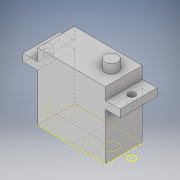
# Autodesk Inventor part: micro_servo
Saved by Autodesk Inventor 2018 (Build 220112000, 112)
## iProperties
Created: 2018-04-21
Part Number: micro_servo
Material: Generic
Document SubType Name: Modeling
Designer: scwu
Density: 1 g/cm^3
Appearance: Default
Author: scwu
Autodesk Inventor part; units mm, degrees
ref_plane "YZ Plane" through (0, 0, 0) normal (1, 0, 0) x (0, 1, 0)
ref_plane "XZ Plane" through (0, 0, 0) normal (0, 1, 0) x (-1, 0, 0)
ref_plane "XY Plane" through (0, 0, 0) normal (0, 0, 1) x (1, 0, 0)
sketch "Sketch1" plane through (0, 0, 0) normal (0, 0, 1) x (1, 0, 0)
  line L0 (-11.25, 0) -> (11.25, 0)
  line L1 (11.25, 0) -> (11.25, 15.72)
  line L2 (11.25, 15.72) -> (16.13, 15.72)
  line L3 (16.13, 15.72) -> (16.13, 18.22)
  line L4 (16.13, 18.22) -> (11.25, 18.22)
  line L5 (11.25, 18.22) -> (11.25, 22.22)
  line L6 (11.25, 22.22) -> (-11.25, 22.22)
  line L7 (-11.25, 22.22) -> (-11.25, 18.22)
  line L8 (-11.25, 18.22) -> (-16.13, 18.22)
  line L9 (-16.13, 18.22) -> (-16.13, 15.72)
  line L10 (-16.13, 15.72) -> (-11.25, 15.72)
  line L11 (-11.25, 0) -> (-11.25, 15.72)
  point P0 (0, 0)
  point P1 (0, 0)
  dimension "d0" = 22.5
  dimension "d1" = 15.72
  dimension "d2" = 4.88
  dimension "d3" = 2.5
  dimension "d4" = 4
  dimension "d5" = 4.88
  constraints: 24 end point, 8 perpendicular, 7 point on line, 1 coincident, 1 horizontal, 1 midpoint
  measures "d0" distance of L0.start L0.end
  measures "d1" distance of L0.end L1.end
  measures "d2" distance of L1.end L2.end
  measures "d3" distance of L2.end L3.end
  measures "d4" distance of L4.end L5.end
  measures "d5" distance of L7.end L8.end
extrude "Extrusion1" add sketch "Sketch1" along normal mid plane 12.23
sketch "Sketch2" plane through (-16.13, 18.22, 6.115) normal (0, 1, 0) x (1, 0, 0)
  line L0 (4.88, 12.23) -> (4.88, 0) projected
  line L1 (27.38, 0) -> (4.88, 0) projected
  line L2 (27.38, 12.23) -> (27.38, 0) projected
  line L3 (4.88, 12.23) -> (27.38, 12.23) projected
  line L4 (27.38, 0) -> (4.88, 0) projected
  line L5 (16.13, 0) -> (16.13, 12.23) construction
  line L6 (4.88, 6.115) -> (27.38, 6.115) construction
  circle A0 centre (2.295, 6.115) radius 1.185
  line L7 (27.38, 6.115) -> (4.88, 6.115) construction
  circle A1 centre (29.965, 6.115) radius 1.185
  point P0 (16.13, 6.115)
  dimension "d8" = 2.37
  dimension "d9" = 27.67
  constraints: 6 end point, 4 midpoint, 3 symmetric about line, 2 centre point, 2 point on line, 1 other
  measures "d8" diameter of A0
  measures "d9" distance of A1.centre A0.centre
sketch "Sketch3" plane through (-11.25, 22.22, 6.115) normal (0, 1, 0) x (1, 0, 0)
  circle A0 centre (18.3104, 6.115) radius 2.1368
  point P0 (11.25, 6.115)
  dimension "d10" = 4.2736
  constraints: 1 centre point
  measures "d10" diameter of A0
extrude "Extrusion2" cut sketch "Sketch2" against normal up to next contours A0 | A1
extrude "Extrusion3" add sketch "Sketch3" along normal blind 3
sketch "Sketch4" plane through (-11.25, 0, 6.115) normal (0, -1, 0) x (1, 0, 0)
  circle A0 centre (-2.585, -6.115) radius 1.185 projected
  circle A1 centre (25.085, -6.115) radius 1.185 projected
  line L0 (22.5, -12.23) -> (22.5, 0) projected
  line L1 (0, 0) -> (22.5, 0) projected
  line L2 (0, 0) -> (0, -12.23) projected
  line L3 (22.5, -12.23) -> (0, -12.23) projected
  line L4 (0, -12.23) -> (0, 0) projected
  line L5 (0, -6.115) -> (22.5, -6.115) construction
  line L6 (11.25, 0) -> (11.25, -12.23) construction
  circle A2 centre (18.3104, -6.115) radius 2.1368 projected
  point P0 (11.25, -6.115)
  constraints: 4 end point, 4 midpoint
body "Solid1"
